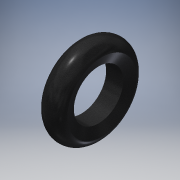
# Autodesk Inventor part: Wheel Tyre
Saved by Autodesk Inventor 2018 (Build 220112000, 112)
## iProperties
Created: 2018-08-07
Part Number: Wheel Tyre
Material: Generic
Document SubType Name: Modeling
Designer: ruben
Density: 1 g/cm^3
Appearance: Black Cast
Author: ruben
Autodesk Inventor part; units mm, degrees
ref_plane "YZ Plane" through (0, 0, 0) normal (1, 0, 0) x (0, 1, 0)
ref_plane "XZ Plane" through (0, 0, 0) normal (0, 1, 0) x (-1, 0, 0)
ref_plane "XY Plane" through (0, 0, 0) normal (0, 0, 1) x (1, 0, 0)
sketch "Sketch1" plane through (0, 0, 0) normal (0, 1, 0) x (-1, 0, 0)
  line L0 (-48.8, 0) -> (-111.45, 0) projected
  line L1 (0, -101.6185) -> (0, 104.2113) projected
  line L2 (-57.75, -20) -> (-57.75, 20)
  line L3 (-57.75, -20) -> (-80.75, -28)
  line L4 (-57.75, 20) -> (-80.75, 28)
  line L5 (-102.5, -72.2142) -> (-102.5, 74.8071) construction
  arc A0 (-80.75, 28) -> (-80.75, -28) centre (-73.602, 0) ccw
  point P0 (-102.5, 0)
  dimension "d0" = 40
  dimension "d1" = 115.5
  dimension "d2" = 23
  dimension "d3" = 23
  dimension "d4" = 8
  dimension "d5" = 8
  dimension "d6" = 205
  constraints: 8 end point, 3 point on circle, 2 point on line, 2 vertical, 1 centre point, 1 parallel, 1 symmetric about line
  measures "d0" distance of L2.end L2.start
  measures "d1" diameter of L2 L1
  measures "d2" horizontal distance of L4.end L2.end
  measures "d3" horizontal distance of L3.end L2.start
  measures "d4" vertical distance of L2.start L3.end
  measures "d5" vertical distance of L2.end L4.end
  measures "d6" diameter of L5 L1
revolve "Revolution1" add sketch "Sketch1" angle 360 about axis through (0, 0, -10) along (0, 0, 1)
equation "\"d2\" = d3"
equation "\"d5\" = d4"
body "Solid1"
